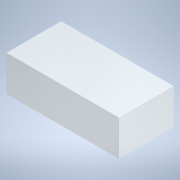
# Autodesk Inventor part: Bateria_14V8
Saved by Autodesk Inventor 2020 (Build 240168000, 168)
## iProperties
Created: 2019-06-28
Part Number: Bateria_14V8
Material: Glass
Document SubType Name: Modeling
Designer: atmat
Density: 2.18 g/cm^3
Appearance: Clear
Mass: 129.424 g
Surface Area: 101.127 cm^2
Volume: 59.3689 cm^3
Author: atmat
Autodesk Inventor part; units mm, degrees
ref_plane "YZ Plane" through (0, 0, 0) normal (1, 0, 0) x (0, 1, 0)
ref_plane "XZ Plane" through (0, 0, 0) normal (0, 1, 0) x (-1, 0, 0)
ref_plane "XY Plane" through (0, 0, 0) normal (0, 0, 1) x (1, 0, 0)
sketch "Szkic1" plane through (0, 0, 0) normal (0, 1, 0) x (-1, 0, 0)
  line L0 (37, 18) -> (-37, 18)
  line L1 (-37, 18) -> (-37, -18)
  line L2 (-37, -18) -> (37, -18)
  line L3 (37, -18) -> (37, 18)
  point P0 (0, 0)
  dimension "d0" = 36
  dimension "d1" = 74
  dimension "d2" = 18
  dimension "d3" = 37
  constraints: 8 end point, 2 parallel, 1 horizontal, 1 perpendicular
  measures "d0" distance of L2.end L0.start
  measures "d1" distance of L1.end L2.end
  measures "d2" distance from line of point (0, 0) L2
  measures "d3" distance from line of L3 point (0, 0)
extrude "Wyciągnięcie proste1" add sketch "Szkic1" along normal blind 23.5
